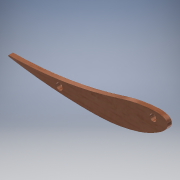
# Autodesk Inventor part: flap_s
Saved by Autodesk Inventor 2018 (Build 220112000, 112)
## iProperties
Created: 2018-03-11
Part Number: flap_s
Material: 木材 (オーク)
Document SubType Name: Modeling
Designer: ku_sk
Density: 0.76 g/cm^3
Appearance: ホワイト オーク材 - ナチュラル 標準の光沢
Author: ku_sk
Autodesk Inventor part; units mm, degrees
ref_plane "YZ Plane" through (0, 0, 0) normal (1, 0, 0) x (0, 1, 0)
ref_plane "XZ Plane" through (0, 0, 0) normal (0, 1, 0) x (-1, 0, 0)
ref_plane "XY Plane" through (0, 0, 0) normal (0, 0, 1) x (1, 0, 0)
sketch "スケッチ1" plane through (0, 0, 0) normal (0, 1, 0) x (-1, 0, 0)
  arc A0 (139.5982, -20.0714) -> (139.3421, -16.8944) centre (139.3282, -18.4944) ccw projected
  arc A1 (72.9436, -26.3461) -> (139.5982, -20.0714) centre (64.9013, 416.2515) ccw projected
  arc A2 (54.0641, -26.1303) -> (72.9436, -26.3461) centre (67.1484, 292.5868) ccw projected
  arc A3 (19.3892, -19.9666) -> (54.0641, -26.1303) centre (59.4352, 104.7024) ccw projected
  arc A4 (-0.6275, -10.135) -> (19.3892, -19.9666) centre (42.8692, 53.13) ccw projected
  arc A5 (-6.31, -4.6171) -> (-0.6275, -10.135) centre (12.76, 9.3368) ccw projected
  arc A6 (-3.299, 4.6397) -> (-6.31, -4.6171) centre (-1.4678, -1.074) ccw projected
  arc A7 (5.2215, 5.7549) -> (-3.299, 4.6397) centre (4.0256, -18.2153) ccw projected
  arc A8 (36.4188, 0) -> (5.2215, 5.7549) centre (-0.7578, -114.096) ccw projected
  arc A9 (36.4188, 0) -> (38.3204, -0.6152) centre (185.125, 456.3841) ccw projected
  arc A10 (38.3204, -0.6152) -> (139.3421, -16.8944) centre (142.307, 323.0926) ccw projected
  point P0 (0, 0)
extrude "押し出し1" add sketch "スケッチ1" along normal mid plane 4
sketch "スケッチ2" plane through (0, -2, 0) normal (0, -1, 0) x (1, 0, 0)
  circle A0 centre (-6.8478, -1.4519) radius 3
  circle A1 centre (-92.934, -19.7045) radius 3
  line L0 (0, 0) -> (-112.4991, -23.8528)
  arc A2 (-139.5982, -20.0714) -> (-72.9436, -26.3461) centre (-64.9013, 416.2515) ccw projected
  dimension "d3" = 6
  dimension "d4" = 6
  dimension "d5" = 115
  dimension "d6" = 7
  dimension "d7" = 95
  constraints: 2 centre point, 2 end point, 2 point on line, 1 point on circle
  measures "d3" diameter of A0
  measures "d4" diameter of A1
  measures "d5" distance of L0.start L0.end
  measures "d6" distance of A0.centre L0.start
  measures "d7" distance of L0.start A1.centre
extrude "押し出し2" cut sketch "スケッチ2" against normal through all
thicken "厚み1" operation cut thickness 1 both sides no extend neighbours no toward (0.0338891, 0, -0.9994256) faces at (-130.7847, 0.6667, -16.7121) (-37.4749, 0.6667, -0.3428) (-8.7492, -0.6667, 5.5268) (2.3792, -0.6667, 4.9143) (6.574, -0.6667, -4.2247) (1.3466, -0.6667, -9.6205) (-17.0344, -0.6667, -19.1679) (-50.1454, -0.6667, -25.9105) (-56.1608, 0.6667, -26.2095) (-102.6817, 0.6667, -24.804) (-139.7269, 0.6667, -20.0439)
